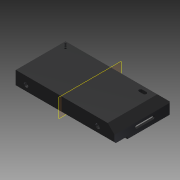
# Autodesk Inventor part: Soporte LCD_CAM Elecfreak
Saved by Autodesk Inventor 2015 (Build 190159000, 159)
## iProperties
Company: MARCHA TECHNOLOGY
Created: 2013-09-30
Part Number: Soporte LCD_CAM Elecfreak
Document SubType Name: Modeling
Designer: O.Martin
Density: 1 g/cm^3
Project: WITBOXprinter_K01
Stock Number: 28655
Description: SOPORTE LCD
Mass: 40.6324 g
Surface Area: 426.774 cm^2
Volume: 40.6324 cm^3
Material: Generic
Appearance: Rubber - Black - Version 1.1
Author: O.Martin
Autodesk Inventor part; units mm, degrees
ref_plane "XZ Plane" through (0, 0, 0) normal (0, 1, 0) x (-1, 0, 0)
ref_plane "XY Plane" through (0, 0, 0) normal (0, 0, 1) x (1, 0, 0)
sketch "Boceto1" plane through (0, 0, 0) normal (0, 0, 1) x (1, 0, 0)
  line L0 (-77.5, 41.5) -> (77.5, 41.5)
  line L1 (77.5, 41.5) -> (77.5, -41.5)
  line L2 (77.5, -41.5) -> (-77.5, -41.5)
  line L3 (-77.5, -41.5) -> (-77.5, 41.5)
  line L4 (-67.5, 36.5) -> (67.5, 36.5)
  line L5 (67.5, 36.5) -> (67.5, -41.5)
  line L6 (67.5, -41.5) -> (-67.5, -41.5)
  line L7 (-67.5, -41.5) -> (-67.5, 36.5)
  line L8 (-72.5, 36.5) -> (72.5, 36.5) construction
  line L9 (72.5, 36.5) -> (72.5, -13.5) construction
  line L10 (72.5, -13.5) -> (-72.5, -13.5) construction
  line L11 (-72.5, -13.5) -> (-72.5, 36.5) construction
  line L12 (67.5, -26.5) -> (-67.5, -26.5)
  line L13 (72.5, -9.2) -> (67.5, -9.2)
  line L14 (67.5, -9.2) -> (67.5, 36.5)
  line L15 (67.5, 36.5) -> (72.5, 36.5)
  line L16 (72.5, 36.5) -> (72.5, -9.2)
  line L17 (-67.5, 36.5) -> (-72.5, 36.5)
  line L18 (-72.5, 36.5) -> (-72.5, -9.2)
  line L19 (-72.5, -9.2) -> (-67.5, -9.2)
  line L20 (-67.5, -9.2) -> (-67.5, 36.5)
  point P0 (0, 0)
  point P1 (0, 41.5)
  point P2 (-77.5, 0)
  point P3 (0, -41.5)
  point P4 (0, 36.5)
  dimension "d0" = 155
  dimension "d1" = 83
  dimension "d3" = 5
  dimension "d4" = 145
  dimension "d5" = 50
  dimension "d6" = 5
  dimension "d44" = 15
  dimension "d160" = 10
  dimension "d161" = 5
  dimension "d162" = 5
  constraints: 42 end point, 10 parallel, 6 perpendicular, 5 horizontal, 5 midpoint, 3 point on line, 2 horizontal alignment, 2 vertical alignment
  measures "d0" distance of L0.start L0.end
  measures "d1" distance of L2.end L0.start
  measures "d3" distance between parallel lines of L0 L4
  measures "d4" distance of L8.start L8.end
  measures "d5" distance of L10.end L8.start
  measures "d6" distance between parallel lines of L0 L8
  measures "d44" distance between parallel lines of L2 L12
  measures "d160" distance between parallel lines of L1 L5
  measures "d161" distance between parallel lines of L1 L16
  measures "d162" distance between parallel lines of L3 L18
extrude "Extrusión1" add sketch "Boceto1" along normal blind 25
chamfer "Chaflán11" distance 10 angle 45 3 edges at (0, 41.5, 25) (77.5, 0, 25) (-77.5, 0, 25)
sketch "Boceto40" plane through (0, 0, 0) normal (0, 0, -1) x (-1, 0, 0)
  line L0 (77.5, 41.5) -> (77.5, -41.5) projected
  line L1 (-77.5, -41.5) -> (-77.5, 41.5) projected
  line L2 (77.5, -41.5) -> (-77.5, -41.5) projected
  line L3 (-77.5, -22.5) -> (77.5, -22.5)
  dimension "d329" = 19
  constraints: 2 end point, 2 point on line, 1 perpendicular
  measures "d329" distance between parallel lines of L2 L3
extrude "Extrusión39" cut sketch "Boceto40" against normal blind 3.5
chamfer "Chaflán13" distance 2 angle 45 1 edges at (0, -41.5, 3.5)
sketch "Boceto41" plane through (-67.5, -41.5, 25) normal (0, -1, 0) x (1, 0, 0)
  line L0 (135, 0) -> (0, 0) projected
  line L1 (-10, -19.5) -> (-10, -10) projected
  line L2 (120, -11.7) -> (15, -11.7) construction
  line L3 (145, -25) -> (-10, -25) construction
  point P0 (67.5, -11.7)
  point P1 (67.5, 0)
  dimension "d335" = 105
  dimension "d336" = 13.3
  constraints: 2 coincident, 2 end point, 2 midpoint, 1 perpendicular, 1 vertical alignment
  measures "d335" distance of L2.start L2.end
  measures "d336" distance between parallel lines of L3 L2
hole "Agujero6" at (52.5, -41.5, 13.3) at (-52.5, -41.5, 13.3) direction (0, 1, 0) diameter 6.647 depth 20 tip angle 118 thread size "M8x1.25" class "6H" standard "ISO Metric profile"
sketch "Boceto42" plane through (0, 0, 0) normal (0, 0, -1) x (-1, 0, 0)
  line L0 (77.5, 41.5) -> (77.5, -22.5) projected
  line L1 (-77.5, 41.5) -> (77.5, 41.5) projected
  line L2 (-77.5, -22.5) -> (-77.5, 41.5) projected
  line L3 (-75.5, 39.5) -> (75.5, 39.5)
  line L4 (75.5, 39.5) -> (75.5, -18.1)
  line L5 (75.5, -18.1) -> (-75.5, -18.1)
  line L6 (-75.5, -18.1) -> (-75.5, 39.5)
  dimension "d345" = 2
  dimension "d346" = 2
  dimension "d347" = 2
  dimension "d362" = 57.6
  constraints: 8 end point, 2 parallel, 1 horizontal, 1 perpendicular
  measures "d345" distance between parallel lines of L3 L1
  measures "d346" distance between parallel lines of L2 L6
  measures "d347" distance between parallel lines of L0 L4
  measures "d362" distance of L5.end L3.start
extrude "Extrusión40" cut sketch "Boceto42" against normal blind 6.8
fillet "Empalme35" radius 2.5 4 edges at (75.5, 39.5, 3.4) (-75.5, 39.5, 3.4) (-75.5, -18.1, 3.4) (75.5, -18.1, 3.4)
sketch "Boceto43" plane through (0, 0, 6.8) normal (0, 0, -1) x (-1, 0, 0)
  line L0 (73, 39.5) -> (-73, 39.5) projected
  line L1 (-72.5, 35.7) -> (72.5, 35.7) construction
  line L2 (72.5, 35.7) -> (72.5, -14.3) construction
  line L3 (72.5, -14.3) -> (-72.5, -14.3) construction
  line L4 (-72.5, -14.3) -> (-72.5, 35.7) construction
  line L5 (-77.5, -41.5) -> (77.5, -41.5) construction
  point P0 (0, 39.5)
  point P1 (0, 35.7)
  dimension "d352" = 145
  dimension "d353" = 50
  dimension "d354" = 27.2
  constraints: 8 end point, 4 coincident, 2 midpoint, 2 parallel, 1 horizontal, 1 perpendicular, 1 vertical alignment
  measures "d352" distance of L1.start L1.end
  measures "d353" distance of L1.end L2.end
  measures "d354" distance between parallel lines of L3 L5
hole "Agujero7" at (72.5, 35.7, 6.8) at (-72.5, 35.7, 6.8) at (-72.5, -14.3, 6.8) at (72.5, -14.3, 6.8) direction (0, 0, 1) diameter 2.459 depth 10 tip angle 118 thread size "M3x0.5" class "6H" standard "ISO Metric profile"
sketch "Boceto44" plane through (0, 0, 0) normal (0, 0, -1) x (-1, 0, 0)
  line L0 (73, -18.1) -> (-73, -18.1) projected
  line L1 (-77.5, -22.5) -> (77.5, -22.5) projected
  line L2 (-77.5, -22.5) -> (-77.5, 41.5) projected
  line L3 (-62.9, -18.1) -> (37.1, -18.1)
  line L4 (37.1, -18.1) -> (37.1, -22.5)
  line L5 (37.1, -22.5) -> (-62.9, -22.5)
  line L6 (-62.9, -22.5) -> (-62.9, -18.1)
  line L7 (-12.9, -18.1) -> (-12.9, -22.5) construction
  dimension "d363" = 64.6
  dimension "d364" = 100
  constraints: 10 end point, 2 midpoint, 2 parallel, 2 point on line, 1 horizontal, 1 perpendicular
  measures "d363" distance between parallel lines of L7 L2
  measures "d364" distance between parallel lines of L4 L6
extrude "Extrusión41" cut sketch "Boceto44" against normal up to surface (3.5 mm away)
sketch "Boceto45" plane through (0, 0, 6.8) normal (0, 0, -1) x (-1, 0, 0)
  circle A0 centre (-72.5, -14.3) radius 1.2295 projected
  circle A1 centre (72.5, 35.7) radius 1.2295 projected
  circle A2 centre (-72.5, 35.7) radius 1.2295 projected
  line L0 (75.5, -15.6) -> (75.5, 37) projected
  line L1 (-75.5, 33.7) -> (74, 33.7)
  line L2 (-75.5, -12.3) -> (74, -12.3)
  line L3 (-75.5, 33.7) -> (-75.5, -12.3)
  line L4 (74, -12.3) -> (74, 33.7)
  line L5 (-75.5, 37) -> (-75.5, -15.6) projected
  dimension "d375" = 1.5
  dimension "d376" = 2
  dimension "d377" = 2
  constraints: 8 end point, 2 vertical, 1 horizontal, 1 perpendicular, 1 point on line
  measures "d375" distance from line of A1.centre L4
  measures "d376" distance from line of L1 A2.centre
  measures "d377" distance from line of A0.centre L2
extrude "Extrusión42" cut sketch "Boceto45" against normal blind 10 contours L1 L4 L2 L3
fillet "Empalme36" radius 5 3 edges at (-74, 33.7, 11.8) (-74, -12.3, 11.8) (75.5, 33.7, 11.8)
fillet "Empalme36" radius 2.5 1 edges at (75.5, -12.3, 11.8)
sketch "Boceto47" plane through (77.5, -41.5, 15) normal (1, 0, 0) x (0, 0, -1)
  line L0 (15, 19) -> (15, 83) projected
  line L1 (9.5, 0) -> (0, 0) projected
  line L2 (5.25, 56.9) -> (7.75, 56.9)
  line L3 (7.75, 56.9) -> (7.75, 32.65)
  line L4 (7.75, 32.65) -> (5.25, 32.65)
  line L5 (5.25, 32.65) -> (5.25, 56.9)
  circle A0 centre (6.5, 32.65) radius 1.25
  circle A1 centre (6.5, 56.9) radius 1.25
  line L6 (8.2, 78.5) -> (8.2, 81) projected
  dimension "d384" = 2.5
  dimension "d388" = 8.5
  dimension "d391" = 24.25
  dimension "d392" = 32.65
  constraints: 8 end point, 2 horizontal alignment, 2 midpoint, 2 parallel, 1 horizontal, 1 perpendicular, 4 other
  measures "d384" distance of L3.end L4.end
  measures "d388" distance from line of point (6.5, 56.9) L0
  measures "d391" distance between parallel lines of L2 L4
  measures "d392" distance between parallel lines of L1 L4
extrude "Extrusión43" cut sketch "Boceto47" against normal blind 10
chamfer "Chaflán14" distance 2 angle 30 4 edges at (77.5, 3.275, 9.75) (77.5, 16.65, 8.5) (77.5, 3.275, 7.25) (77.5, -10.1, 8.5) measured on face at (77, -10.1, 8.5) measured on face at (77, 3.275, 7.25) measured on face at (77, 3.275, 9.75) measured on face at (77, 16.65, 8.5)
sketch "Boceto48" plane through (-77.5, -41.5, 15) normal (-1, 0, 0) x (0, 0, 1)
  line L0 (-9.5, 0) -> (0, 0) projected
  line L1 (-15, 83) -> (-15, 19) projected
  line L2 (-15, 50) -> (-3, 50)
  line L3 (-3, 50) -> (-3, 30)
  line L4 (-3, 30) -> (-15, 30)
  line L5 (-15, 30) -> (-15, 50)
  dimension "d396" = 50
  dimension "d397" = 20
  dimension "d398" = 12
  constraints: 8 end point, 2 parallel, 1 horizontal, 1 perpendicular, 1 point on line
  measures "d396" distance between parallel lines of L0 L2
  measures "d397" distance of L2.end L3.end
  measures "d398" distance of L2.start L2.end
extrude "Extrusión44" cut sketch "Boceto48" against normal blind 10
sketch "Boceto49" plane through (0, 0, 25) normal (0, 0, 1) x (1, 0, 0)
  line L0 (50.5, 26.5) -> (56.5, 26.5)
  line L1 (56.5, 26.5) -> (56.5, 21.5)
  line L2 (56.5, 21.5) -> (50.5, 21.5)
  line L3 (50.5, 21.5) -> (50.5, 26.5)
  circle A0 centre (50.5, 24) radius 2.5
  circle A1 centre (56.5, 24) radius 2.5
  line L4 (67.5, -41.5) -> (-67.5, -41.5) projected
  line L5 (77.5, -41.5) -> (77.5, 41.5) projected
  dimension "d401" = 5
  dimension "d402" = 6
  dimension "d405" = 65.5
  dimension "d406" = 21
  constraints: 8 end point, 2 midpoint, 2 parallel, 2 vertical alignment, 1 horizontal, 1 perpendicular, 4 other
  measures "d401" distance of L0.end L1.end
  measures "d402" distance of L0.start L0.end
  measures "d405" distance from line of L4 point (56.5, 24)
  measures "d406" distance between parallel lines of L5 L1
extrude "Extrusión45" cut sketch "Boceto49" against normal through all
sketch "Boceto50" plane through (0, 0, 3.5) normal (0, 0, -1) x (-1, 0, 0)
  line L0 (77.5, -22.5) -> (77.5, -39.5) projected
  line L1 (-77.5, -41.5) -> (77.5, -41.5) projected
  line L2 (77.5, -41.5) -> (67.5, -41.5)
  line L3 (67.5, -41.5) -> (67.5, -31.5)
  line L4 (67.5, -31.5) -> (77.5, -31.5)
  line L5 (77.5, -31.5) -> (77.5, -41.5)
  dimension "d407" = 10
  dimension "d408" = 10
  constraints: 8 end point, 2 parallel, 1 horizontal, 1 perpendicular
  measures "d407" distance between parallel lines of L0 L3
  measures "d408" distance between parallel lines of L1 L4
extrude "Extrusión46" cut sketch "Boceto50" against normal through all
fillet "Empalme37" radius 5 1 edges at (-67.5, -31.5, 14.25)
chamfer "Chaflán15" distance 2 angle 45 2 edges at (-77.5, 41.5, 7.5) (77.5, 41.5, 7.5)
sketch "Boceto51" plane through (0, 0, 16.8) normal (0, 0, -1) x (-1, 0, 0)
  arc A0 (-70.5, 33.7) -> (-75.5, 28.7) centre (-70.5, 28.7) ccw projected
  line L0 (-75.5, 28.7) -> (-75.5, -9.8) projected
  arc A1 (-75.5, -9.8) -> (-73, -12.3) centre (-73, -9.8) ccw projected
  line L1 (-73, -12.3) -> (69, -12.3) projected
  line L2 (69, 33.7) -> (-70.5, 33.7) projected
  line L3 (-70.5, 28.7) -> (-70.5, -7.3)
  arc A2 (-65.5, 33.7) -> (-70.5, 28.7) centre (-65.5, 28.7) ccw
  arc A3 (-70.5, -7.3) -> (-65.5, -12.3) centre (-65.5, -7.3) ccw
  line L4 (74, -7.3) -> (74, 28.7) projected
  line L5 (69, -7.3) -> (69, 28.7)
  arc A4 (69, 28.7) -> (64, 33.7) centre (64, 28.7) ccw
  arc A5 (64, -12.3) -> (69, -7.3) centre (64, -7.3) ccw
  arc A6 (69, -12.3) -> (74, -7.3) centre (69, -7.3) ccw projected
  arc A7 (74, 28.7) -> (69, 33.7) centre (69, 28.7) ccw projected
  dimension "d416" = 5
  dimension "d419" = 5
  constraints: 8 point on circle, 8 tangent, 4 centre point, 4 end point, 4 equal radius, 4 point on line, 1 parallel, 1 perpendicular
  measures "d416" distance between parallel lines of L0 L3
  measures "d419" distance between parallel lines of L4 L5
extrude "Extrusión47" add sketch "Boceto51" along normal up to surface (4.8 mm away) contours L2 A2 L3 A3 L1 A1 L0 A0 | L2 A7 L4 A6 L1 A5 L5 A4
sketch "Boceto52" plane through (0, 0, 16.8) normal (0, 0, -1) x (-1, 0, 0)
  arc A0 (-70.5, -7.3) -> (-65.5, -12.3) centre (-65.5, -7.3) ccw projected
  line L0 (-65.5, -12.3) -> (64, -12.3) projected
  arc A1 (64, -12.3) -> (69, -7.3) centre (64, -7.3) ccw projected
  line L1 (69, -7.3) -> (69, 28.7) projected
  arc A2 (69, 28.7) -> (64, 33.7) centre (64, 28.7) ccw projected
  line L2 (64, 33.7) -> (-65.5, 33.7) projected
  arc A3 (-65.5, 33.7) -> (-70.5, 28.7) centre (-65.5, 28.7) ccw projected
  line L3 (-70.5, 28.7) -> (-70.5, -7.3) projected
  line L4 (-56.5, 26.5) -> (-50.5, 26.5) projected
  arc A4 (-50.5, 21.5) -> (-50.5, 26.5) centre (-50.5, 24) ccw projected
  line L5 (-50.5, 21.5) -> (-56.5, 21.5) projected
  arc A5 (-56.5, 26.5) -> (-56.5, 21.5) centre (-56.5, 24) ccw projected
extrude "Extrusión48" cut sketch "Boceto52" against normal blind 2
sketch "Boceto55" plane through (0, 0, 25) normal (0, 0, 1) x (1, 0, 0)
  line L0 (-67.5, 31.5) -> (67.5, 31.5) projected
  line L1 (-67.5, 31.5) -> (-58.5, 22.5) construction
  point P0 (-61.3284, 25.3284)
  point P1 (-64.1569, 28.1569)
  dimension "d444" = 45
  dimension "d445" = 4
  dimension "d446" = 9
  dimension "d454" = 4
  dimension "d177" = 145
  dimension "d178" = 50
  dimension "d283" = 3
  dimension "d285" = 5
  dimension "d207" = 47.9
  dimension "d208" = 80
  dimension "d209" = 13.5
  dimension "d210" = 12
  dimension "d229" = 12
  constraints: 2 end point, 2 point on line, 1 coincident
  measures "d444" angle of L0 L1
  measures "d445" distance of point (-61.328, 25.328) point (-58.5, 22.5)
  measures "d446" horizontal distance of L0.start L1.end
  measures "d454" distance of point (-61.328, 25.328) point (-64.157, 28.157)
hole "Agujero10" at (-58.5, 22.5, 25) at (-61.3284, 25.3284, 25) at (-64.1569, 28.1569, 25) direction (0, 0, -1) diameter 2.5 depth 8 tip angle 118
sketch "Boceto28" plane through (-75, -41.05, 0) normal (0, -1, 0) x (1, 0, 0)
  circle A0 centre (47.9, 6.5) radius 3.125 projected
  line L0 (0, 0) -> (0, 10) projected
  line L1 (0, 0) -> (150, 0) projected
  line L2 (150, 0) -> (150, 10) projected
  arc A1 (41.4, 6.5) -> (47.9, 0) centre (47.9, 6.5) ccw
  line L3 (41.4, 6.5) -> (41.4, 10)
  line L4 (41.4, 10) -> (0, 10)
  constraints: 4 end point, 2 point on circle, 2 tangent, 1 centre point, 1 coincident, 1 parallel, 1 point on line
sketch "Boceto29" plane through (0, 0, 0) normal (0, 0, -1) x (-1, 0, 0)
  line L0 (-75, -41.05) -> (-75, 41.05) projected
  line L1 (-75, -11.5) -> (-70.8518, -11.5)
  line L2 (-70.8518, -11.5) -> (-70.8518, 18.5)
  line L3 (-70.8518, 18.5) -> (-75, 18.5)
  line L4 (-75, 18.5) -> (-75, -11.5)
  line L5 (-75, 41.05) -> (75, 41.05) projected
  dimension "d254" = 30
  dimension "d286" = 22.55
  dimension "d267" = 17.5
  dimension "d268" = 10
  dimension "d271" = 2
  constraints: 10 end point, 4 point on circle, 3 tangent, 2 centre point, 2 point on line, 1 collinear, 1 parallel, 1 vertical, 3 other
sketch "Boceto34" plane through (0, 0, 25) normal (0, 0, 1) x (1, 0, 0)
  circle A0 centre (72.5, 36.05) radius 1.5 projected
  circle A1 centre (57, 24.55) radius 2.5
  line L0 (-62.5, -41.05) -> (-63.7574, -41.05) projected
  circle A2 centre (51, 24.55) radius 2.5
  line L1 (51, 27.05) -> (57, 27.05)
  line L2 (51, 22.05) -> (57, 22.05)
  dimension "d306" = 15.5
  dimension "d307" = 11.5
  dimension "d308" = 5
  dimension "d328" = 6
  constraints: 4 end point, 4 point on circle, 3 tangent, 2 centre point, 1 equal radius, 1 horizontal alignment, 1 parallel
  measures "d306" horizontal distance of A0.centre A1.centre
  measures "d307" vertical distance of A0.centre A1.centre
  measures "d308" diameter of A1
  measures "d328" distance of A1.centre A2.centre
sketch "Boceto37" plane through (64.5029, 30.5529, 10.703) normal (0, 0, -1) x (-1, 0, 0)
  line L0 (137.1029, 2.4971) -> (137.0029, 2.4971) construction
  arc A0 (134.039, 5.0331) -> (137.0029, 2.4971) centre (137.0029, 5.4971) ccw construction
  line L1 (129.0059, 0) -> (134.039, 5.0331) construction
  line L2 (129.0059, -69.2029) -> (129.0059, 0) construction
  line L3 (137.1029, -69.2029) -> (129.0059, -69.2029) construction
  line L4 (137.1029, -47.5029) -> (137.1029, -69.2029) construction
  line L5 (137.1029, -47.5029) -> (137.0029, -47.5029) construction
  arc A1 (137.0029, -41.5029) -> (137.0029, -47.5029) centre (137.0029, -44.5029) ccw construction
  line L6 (137.0029, -41.5029) -> (137.1029, -41.5029) construction
  line L7 (137.1029, 2.4971) -> (137.1029, -41.5029) construction
  line L8 (-4.9971, 8.0971) -> (-4.9971, 5.4971) construction
  arc A2 (-5.0331, 5.0331) -> (-4.9971, 5.4971) centre (-7.9971, 5.4971) ccw construction
  line L9 (-5.0331, 5.0331) -> (0, 0) construction
  line L10 (129.0059, 0) -> (0, 0) construction
  line L11 (129.0059, 0) -> (134.039, 5.0331) construction
  arc A3 (134.0029, 5.4971) -> (134.039, 5.0331) centre (137.0029, 5.4971) ccw construction
  line L12 (134.0029, 5.4971) -> (134.0029, 8.0971) construction
  line L13 (-4.9971, 8.0971) -> (134.0029, 8.0971) construction
  line L14 (-6.0971, -42.1813) -> (-6.0971, 3.1754) construction
  line L15 (88.4779, -56.6029) -> (94.7279, -56.6029) projected
  arc A4 (-7.9971, 5.4971) -> (137.0029, 5.4971) centre (64.5029, 37.6079) ccw
  line L16 (5.6029, -56.6029) -> (17.6029, -56.6029) projected
  line L17 (85.6029, -56.6029) -> (97.6029, -56.6029) projected
  line L18 (8.4779, -56.6029) -> (14.7279, -56.6029) projected
  arc A5 (97.6029, -56.6029) -> (5.6029, -56.6029) centre (51.6029, -56.6029) ccw
  arc A6 (-5.1744, 6.5328) -> (134.4815, 7.217) centre (64.5029, 37.6079) ccw
  line L19 (-7.9971, 5.4971) -> (-5.1744, 6.5328)
  line L20 (134.4815, 7.217) -> (137.0029, 5.4971)
  line L21 (85.6029, -69.2029) -> (85.6029, -56.6029) construction
  arc A7 (94.6029, -56.6029) -> (8.6029, -56.6029) centre (51.6029, -56.6029) ccw
  line L22 (94.6029, -56.6029) -> (97.6029, -56.6029)
  line L23 (8.6029, -56.6029) -> (5.6029, -56.6029)
  dimension "d316" = 3
  dimension "d320" = 3
  constraints: 8 end point, 8 point on circle, 4 centre point, 2 point on line, 1 collinear, 1 perpendicular, 2 other
  measures "d316" radial gap between concentric circles of A4 A6
  measures "d320" radial gap between concentric circles of A5 A7
sketch "Boceto38" plane through (64.5029, 30.5529, 10.703) normal (0, 0, -1) x (-1, 0, 0)
  arc A0 (13.5029, -8.5029) -> (13.5029, -3.5029) centre (13.5029, -6.0029) ccw projected
  line L0 (7.5029, -3.5029) -> (13.5029, -3.5029) projected
  arc A1 (7.5029, -3.5029) -> (7.5029, -8.5029) centre (7.5029, -6.0029) ccw projected
  line L1 (13.5029, -8.5029) -> (7.5029, -8.5029) projected
  arc A2 (13.5029, -10.526) -> (13.5029, -1.4799) centre (13.5029, -6.0029) ccw
  line L2 (13.5029, -10.526) -> (7.5029, -10.526)
  arc A3 (7.5029, -1.4799) -> (7.5029, -10.526) centre (7.5029, -6.0029) ccw
  line L3 (7.5029, -1.4799) -> (13.5029, -1.4799)
  arc A4 (-4.9971, 6.1381) -> (17.9295, -22.8199) centre (64.5029, 37.6079) ccw projected
  constraints: 4 end point, 4 point on circle, 2 centre point, 1 tangent, 3 other
body "Solid1"
